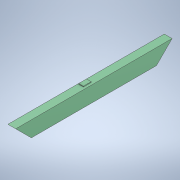
# Autodesk Inventor part: PerfilH1
Saved by Autodesk Inventor 2021 (Build 250183000, 183)
## iProperties
Created: 2021-06-11
Part Number: PerfilH1
Material: Generic
Document SubType Name: Modeling
Designer: lcper
Density: 1 g/cm^3
Appearance: Default
Author: lcper
Autodesk Inventor part; units mm, degrees
ref_plane "YZ Plane" through (0, 0, 0) normal (1, 0, 0) x (0, 1, 0)
ref_plane "XZ Plane" through (0, 0, 0) normal (0, 1, 0) x (-1, 0, 0)
ref_plane "XY Plane" through (0, 0, 0) normal (0, 0, 1) x (1, 0, 0)
sketch "Sketch2" plane through (0, 0, 0) normal (0, 0, 1) x (1, 0, 0)
  line L0 (-9.4777, 15.0257) -> (40.5223, 15.0257)
  line L1 (40.5223, 15.0257) -> (40.5223, -84.9743)
  line L2 (40.5223, -84.9743) -> (-9.4777, -84.9743)
  line L3 (-9.4777, -84.9743) -> (-9.4777, 15.0257)
  line L4 (35.5223, 10.0257) -> (-4.4777, 10.0257)
  line L5 (-4.4777, 10.0257) -> (-4.4777, -79.9743)
  line L6 (-4.4777, -79.9743) -> (35.5223, -79.9743)
  line L7 (35.5223, -79.9743) -> (35.5223, 10.0257)
  point P0 (0, 0)
  point P1 (0, 0)
  dimension "d6" = 50
  dimension "d7" = 100
  dimension "d8" = 5
  dimension "d9" = 90
  dimension "d10" = 5
  dimension "d11" = 40
  constraints: 16 end point, 4 parallel, 2 horizontal, 2 perpendicular
  measures "d6" distance of L1.end L2.end
  measures "d7" distance of L0.end L1.end
  measures "d8" distance between parallel lines of L4 L0
  measures "d9" distance of L6.end L4.start
  measures "d10" distance between parallel lines of L1 L7
  measures "d11" distance of L5.end L6.end
extrude "Extrusion1" add sketch "Sketch2" along normal blind 1000
sketch "Sketch3" plane through (40.5223, -84.9743, 0) normal (1, 0, 0) x (0, 0, -1)
  line L0 (0, 100) -> (-100, 0)
  line L1 (0, 100) -> (141.4214, 100) construction
  line L2 (0, 0) -> (0, 100) projected
  line L3 (0, 100) -> (0, 0)
  line L4 (0, 0) -> (-100, 0)
  line L5 (0, 0) -> (-1000, 0) projected
  line L6 (0, 100) -> (-1000, 100) projected
  line L7 (-1000, 100) -> (-900, 0)
  line L8 (-1000, 100) -> (-858.5786, 100) construction
  line L9 (-1000, 100) -> (-1000, 0)
  line L10 (-1000, 0) -> (-900, 0)
  point P0 (0, 84.9743)
  dimension "d14" = 135
  dimension "d15" = 45
  constraints: 16 end point, 2 equal length, 2 horizontal, 2 vertical, 1 collinear, 1 point on line
  measures "d14" angle of L0 L1
  measures "d15" angle of L7 L8
extrude "Extrusion2" cut sketch "Sketch3" against normal blind 1000 contours L2 L4 L0 | L7 L5 L9
sketch "Sketch5" plane through (-9.4777, 15.0257, 0) normal (0, 1, 0) x (1, 0, 0)
  line L0 (5, -552.5) -> (35.1644, -552.5)
  line L1 (35.1644, -552.5) -> (35.1644, -502.5)
  line L2 (35.1644, -502.5) -> (5, -502.5)
  line L3 (5, -502.5) -> (5, -552.5)
  line L4 (0, 0) -> (0, -1000) projected
  line L5 (50, 0) -> (0, 0) projected
  point P0 (9.4777, 0)
  dimension "d23" = 5
  dimension "d24" = 50
  dimension "d25" = 502.5
  constraints: 8 end point, 2 parallel, 1 horizontal, 1 perpendicular
  measures "d23" distance between parallel lines of L4 L3
  measures "d24" distance of L2.end L0.start
  measures "d25" distance between parallel lines of L5 L2
extrude "Extrusion4" add sketch "Sketch5" along normal blind 5
body "Solid1"
